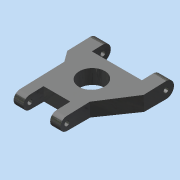
# Autodesk Inventor part: Transmission Plate - Bottom
Saved by Autodesk Inventor 2013 (Build 170138000, 138)
## iProperties
Created: 2011-09-22
Part Number: Transmission Plate - Bottom
Document SubType Name: Modeling
Designer: dgitz
Density: 1 g/cm^3
Material: Generic
d0: 0.310 in
d1: 0.115 in
d2: 0.370 in
d3: 0.115 in
d4: 2.160 in
d5: 1.800 in
d6: 0.00 deg
d10: 0.230 in
d12: 0.630 in
d14: 1.200 in
d16: 0.310 in
d17: 0.440 in
d18: 0.480 in
d20: 0.00 deg
d21: 1.450 in
d22: 0.240 in
d24: 0.700 in
d25: 0.610 in
d26: 0.240 in
d27: 0.370 in
d28: 1.180 in
d29: 0.180 in
Author: dgitz
Autodesk Inventor part; units mm, degrees
ref_plane "YZ Plane" through (0, 0, 0) normal (1, 0, 0) x (0, 1, 0)
sketch "Sketch2" plane through (0, 0, 0) normal (1, 0, 0) x (0, 1, 0)
  arc A0 (11.6091, 219.5578) -> (3.7373, 219.428) centre (7.6743, 219.428) ccw
  circle A1 centre (7.6743, 219.428) radius 1.4605
  arc A2 (3.7373, 173.2) -> (13.1327, 173.3549) centre (8.4363, 173.2) ccw
  circle A3 centre (8.4363, 173.2) radius 1.4605
  line L0 (3.7373, 219.428) -> (3.7373, 173.2)
  line L1 (39.8145, 223.365) -> (24.6856, 223.365) construction
  line L2 (42.3544, 168.501) -> (22.3114, 168.501) construction
  line L3 (11.6091, 219.5578) -> (13.1327, 173.3549)
  point P0 (0, 0)
  point P1 (32.3329, 168.501)
  dimension "d0" = 7.874
  dimension "d1" = 2.921
  dimension "d2" = 9.398
  dimension "d3" = 2.921
  dimension "d4" = 54.864
  constraints: 8 end point, 6 tangent, 4 centre point, 4 point on circle, 2 coincident, 2 horizontal, 1 midpoint, 1 vertical
  measures "d0" diameter of A0
  measures "d1" diameter of A1
  measures "d2" diameter of A2
  measures "d3" diameter of A3
  measures "d4" distance between parallel lines of L2 L1
extrude "Extrusion1" add sketch "Sketch2" along normal mid plane 45.72
sketch "Sketch3" plane through (-22.86, 13.1327, 173.3549) normal (0, 0.9994567, 0.0329581) x (1, 0, 0)
  line L0 (0, 0) -> (0, -46.228) projected
  line L1 (0, -50.165) -> (45.72, -50.165) projected
  line L2 (0, 4.699) -> (45.72, 4.699) projected
  line L3 (45.72, 4.699) -> (45.72, -0.1549) projected
  line L4 (0, -0.1549) -> (0, 4.699) projected
  line L5 (0, -50.165) -> (0, -46.228) projected
  line L6 (10.414, -50.165) -> (26.416, -50.165)
  line L7 (26.416, -50.165) -> (26.416, -37.973)
  line L8 (26.416, -37.973) -> (10.414, -37.973)
  line L9 (10.414, -37.973) -> (10.414, -50.165)
  line L10 (0, -50.165) -> (0, -13.335)
  line L11 (0, -13.335) -> (4.572, -19.685)
  line L12 (4.572, -19.685) -> (4.572, -50.165)
  line L13 (4.572, -50.165) -> (0, -50.165)
  line L14 (47.5768, -13.335) -> (-11.8241, -13.335) construction
  line L15 (7.874, 4.699) -> (37.846, 4.699)
  line L16 (37.846, 4.699) -> (37.846, -6.477)
  line L17 (37.846, -6.477) -> (7.874, -6.477)
  line L18 (7.874, -6.477) -> (7.874, 4.699)
  line L19 (45.72, -46.228) -> (45.72, 0) projected
  line L20 (45.72, -13.335) -> (45.72, -50.165)
  line L21 (45.72, -50.165) -> (32.512, -50.165)
  line L22 (32.512, -50.165) -> (32.512, -32.385)
  line L23 (32.512, -32.385) -> (45.72, -13.335)
  circle A0 centre (21.717, -20.32) radius 7.747
  line L24 (13.97, -14.4458) -> (13.97, -24.81) construction
  line L25 (12.0083, -12.573) -> (20.6899, -12.573) construction
  point P0 (22.86, 172.8279)
  point P1 (0, -46.3578)
  dimension "d10" = 5.842
  dimension "d12" = 16.002
  dimension "d14" = 30.48
  dimension "d16" = 7.874
  dimension "d17" = 11.176
  dimension "d18" = 12.192
  dimension "d21" = 36.83
  dimension "d22" = 6.096
  dimension "d24" = 17.78
  dimension "d25" = 15.494
  dimension "d26" = 6.096
  dimension "d27" = 9.398
  dimension "d28" = 29.972
  dimension "d29" = 4.572
  constraints: 38 end point, 9 point on line, 6 parallel, 6 perpendicular, 2 horizontal, 2 tangent, 1 centre point, 1 collinear
  measures "d10" distance between parallel lines of L9 L12
  measures "d12" distance between parallel lines of L7 L9
  measures "d14" distance of L12.end L11.end
  measures "d16" distance between parallel lines of L4 L18
  measures "d17" distance between parallel lines of L17 L2
  measures "d18" distance between parallel lines of L8 L1
  measures "d21" distance of L1.end L20.start
  measures "d22" distance between parallel lines of L22 L7
  measures "d24" distance from line of L1 L22.end
  measures "d25" diameter of A0
  measures "d26" distance between parallel lines of L25 L17
  measures "d27" distance between parallel lines of L24 L12
  measures "d28" distance between parallel lines of L16 L18
  measures "d29" distance between parallel lines of L12 L10
extrude "Extrusion2" cut sketch "Sketch3" against normal through all contours L11 L12 L1 L5 L0 | L2 L16 L17 L18 | L9 L8 L7 L1 | L22 L23 L19 L20 L1 | A0
ref_plane "Work Plane1" through (0, 7.6743, 223.365) normal (0, 0, 1) x (1, 0, 0)
ref_plane "Work Plane2" through (0, 8.4363, 168.501) normal (0, 0, 1) x (1, 0, 0)
body "Solid1"
